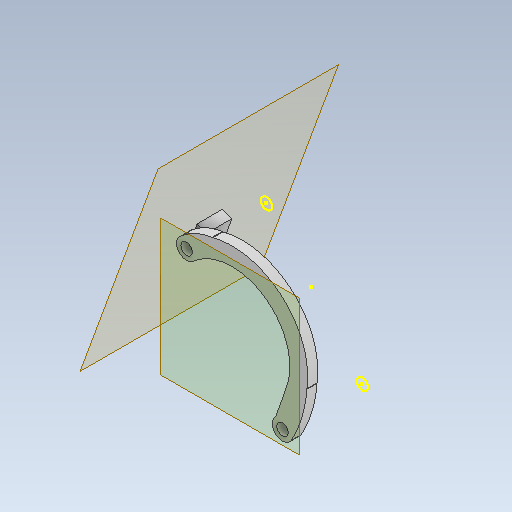
# Autodesk Inventor part: Rear Fan Support
Saved by Autodesk Inventor 2020 (Build 240168000, 168)
## iProperties
Created: 2019-09-23
Part Number: Rear Fan Support
Material: Generic
Document SubType Name: Modeling
Designer: pepd9
Density: 1 g/cm^3
Appearance: Default
Author: pepd9
Autodesk Inventor part; units mm, degrees
ref_plane "YZ Plane" through (0, 0, 0) normal (1, 0, 0) x (0, 1, 0)
ref_plane "XZ Plane" through (0, 0, 0) normal (0, 1, 0) x (-1, 0, 0)
ref_plane "XY Plane" through (0, 0, 0) normal (0, 0, 1) x (1, 0, 0)
sketch "Sketch1" plane through (0, 0, 0) normal (0, 0, 1) x (1, 0, 0)
  circle A0 centre (-18, 20) radius 2.25 projected
  circle A1 centre (20, -23) radius 2.25 projected
  point P0 (0, 0)
ref_plane "Work Plane1" through (-16.0715, 39.2438, 18) normal (0.9396926, -0.3420201, 0) x (0, 0, -1)
sketch "Sketch2" plane through (-16.0715, 39.2438, 18) normal (0.9396926, -0.3420201, 0) x (0, 0, -1)
  circle A0 centre (0, -22.1459) radius 1.8 projected
  line L0 (-5, -26.1459) -> (5, -26.1459)
  line L1 (5, -26.1459) -> (5, -18.1459)
  line L2 (5, -18.1459) -> (-5, -18.1459)
  line L3 (-5, -18.1459) -> (-5, -26.1459)
  line L4 (-5, -26.1459) -> (5, -18.1459) construction
  line L5 (5, -26.1459) -> (-5, -18.1459) construction
  point P0 (18, -31.3803)
  dimension "d0" = 10
  dimension "d1" = 8
  constraints: 12 end point, 2 midpoint, 2 parallel, 1 horizontal, 1 perpendicular
  measures "d0" distance of L2.end L1.end
  measures "d1" distance of L1.end L0.end
extrude "Extrusion1" add sketch "Sketch2" along normal blind 4
ref_plane "Work Plane2" through (0, 0, 31.5) normal (0, 0, -1) x (-1, 0, 0)
sketch "Sketch3" plane through (0, 0, 31.5) normal (0, 0, -1) x (-1, 0, 0)
  circle A0 centre (-20, -23) radius 2.25 projected
  circle A1 centre (18, 20) radius 2.25 projected
  circle A2 centre (-20, -23) radius 4
  circle A3 centre (18, 20) radius 4
  circle A4 centre (0, 0) radius 22.9072
  arc A5 (-21.6886, -7.3719) -> (-17.2648, -20.0813) centre (849.6627, 288.7979) ccw
  circle A6 centre (0, 0) radius 30
  arc A7 (-29.6926, -4.2838) -> (-23.3072, -25.25) centre (20.1636, -0.5552) ccw
  arc A8 (21.4078, 22.0945) -> (7.7375, 28.985) centre (4.6374, 5.8289) ccw
  point P0 (15.3241, 17.0268)
  point P1 (18, 24)
  point P2 (19.8909, 23.5248)
  dimension "d5" = 8
  dimension "d4" = 8
  dimension "d6" = 60
  constraints: 10 point on circle, 5 centre point, 4 coincident, 7 other
  measures "d4" diameter of A2
  measures "d6" diameter of A6
extrude "Extrusion2" add sketch "Sketch3" along normal blind 4 contours A0 A6 A2 | A0 A6 A2 A7 | A6 A3 A4 A5 A2 | A2 A7 A6 | A8 A3 A6 | A6 A3 A8 | A3 A6 | A3 A8 picked at (4.6408, 27.0507)
fillet "Fillet1" radius 3 5 edges at (-19.8909, 23.5248, 29.5) (-7.7375, 28.985, 29.5) (23.3072, -25.25, 29.5) (17.2648, -20.0813, 29.5) (29.6926, -4.2838, 29.5)
body "Solid1"
